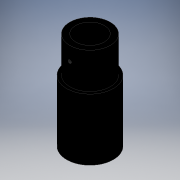
# Autodesk Inventor part: tubus lense (423606-8031)
Saved by Autodesk Inventor 2017 (Build 210142000, 142)
## iProperties
Part Number: tubus lense (423606-8031)
Material: Generisch
Document SubType Name: Modeling
Designer: ExCISS
Density: 1 g/cm^3
Appearance: Eloxiert - schwarz
Author: ExCISS
Autodesk Inventor part; units mm, degrees
note: some values were not read from the file. Chosen so that the rebuilt part matches the saved one: direction of "Bohrung1".
ref_plane "YZ Plane" through (0, 0, 0) normal (1, 0, 0) x (0, 1, 0)
ref_plane "XY Plane" through (0, 0, 0) normal (0, 0, 1) x (1, 0, 0)
sketch "Skizze1" plane through (0, 0, 0) normal (0, 0, 1) x (1, 0, 0)
  circle A0 centre (0, 0) radius 15
  dimension "d0" = 30
  constraints: 1 centre point, 1 coincident
  measures "d0" diameter of A0
extrude "Extrusion1" add sketch "Skizze1" along normal blind 39.6
sketch "Skizze2" plane through (0, 0, 39.6) normal (0, 0, 1) x (1, 0, 0)
  circle A0 centre (0, 0) radius 13
  dimension "d3" = 26
  constraints: 1 centre point, 1 coincident
  measures "d3" diameter of A0
extrude "Extrusion2" add sketch "Skizze2" along normal blind 23
sketch "Skizze5" plane through (0, 0, 62.6) normal (0, 0, 1) x (1, 0, 0)
  circle A0 centre (0, 0) radius 9.2
  dimension "d6" = 18.4
  constraints: 1 centre point, 1 coincident
  measures "d6" diameter of A0
extrude "Extrusion3" cut sketch "Skizze5" against normal through all
sketch "Skizze6" plane through (0, 0, 0) normal (0, 0, -1) x (-1, 0, 0)
  circle A0 centre (0, 0) radius 13.9
  dimension "d9" = 27.8
  constraints: 1 centre point, 1 coincident
  measures "d9" diameter of A0
extrude "Extrusion4" cut sketch "Skizze6" against normal blind 20
ref_plane "Arbeitsebene1" through (0, -13, 39.6) normal (0, 1, 0) x (-1, 0, 0)
sketch "Skizze7" plane through (0, -13, 39.6) normal (0, 1, 0) x (-1, 0, 0)
  line L0 (13, 23) -> (-13, 23) projected
  line L1 (-9.2, 23) -> (9.2, 23) construction
  line L2 (0, 23) -> (0, 14) construction
  point P0 (0, -39.6)
  dimension "d12" = 9
  constraints: 2 end point, 1 coincident, 1 midpoint, 1 vertical
  measures "d12" distance of L2.start L2.end
hole "Bohrung1" at (0, -13, 53.6) direction (0, 1, 0) diameter 2.013 end up to surface thread size "M2.5x0.45" class "6H" standard "ISO Metric profile"
